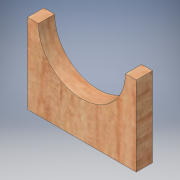
# Autodesk Inventor part: Soporte para Cañón
Saved by Autodesk Inventor 2016 SP2 (Build 200236200, 236)
## iProperties
Created: 2017-06-02
Part Number: Soporte para Cañón
Material: Abedul
Document SubType Name: Modeling
Designer: ssant
Density: 0.512 g/cm^3
Appearance: Abedul - Natural brillo medio
Author: ssant
Autodesk Inventor part; units mm, degrees
ref_plane "YZ Plane" through (0, 0, 0) normal (1, 0, 0) x (0, 1, 0)
ref_plane "XZ Plane" through (0, 0, 0) normal (0, 1, 0) x (-1, 0, 0)
ref_plane "XY Plane" through (0, 0, 0) normal (0, 0, 1) x (1, 0, 0)
sketch "Boceto3" plane through (0, 0, 0) normal (0, 0, 1) x (1, 0, 0)
  line L0 (-30, 22) -> (-30, -22)
  line L1 (-30, -22) -> (30, -22)
  line L2 (30, -22) -> (30, 22)
  line L3 (30, 22) -> (24, 22)
  line L4 (-30, 22) -> (-24, 22)
  arc A0 (-24, 22) -> (24, 22) centre (0, 22) ccw
  point P0 (0, 0)
  point P1 (0, -22)
  point P2 (30, 0)
  dimension "d14" = 44
  dimension "d16" = 60
  dimension "d17" = 44
  dimension "d18" = 6
  dimension "d19" = 6
  dimension "d20" = 90
  dimension "d21" = 48
  constraints: 10 end point, 2 midpoint, 2 perpendicular, 2 point on circle, 1 centre point, 1 horizontal, 1 horizontal alignment, 1 vertical, 1 vertical alignment
  measures "d14" distance of L0.start L0.end
  measures "d16" distance of L0.end L1.end
  measures "d17" distance of L1.end L2.end
  measures "d18" distance of L2.end L3.end
  measures "d19" distance of L0.start L4.end
  measures "d20" angle of L0 L4
  measures "d21" diameter of A0
extrude "Extrusión1" add sketch "Boceto3" against normal blind 9
sketch "Boceto4" plane through (-30, -22, 0) normal (0, -1, 0) x (1, 0, 0)
  line L0 (0, 0) -> (60, 0) projected
  line L1 (0, 0) -> (0, -9) projected
  line L2 (60, -9) -> (0, -9) projected
  line L3 (60, 0) -> (60, -9) projected
  line L4 (60, 0) -> (60, -9) projected
  point P0 (30, 0)
  point P1 (52.5, -4.5)
  point P2 (7.5, -4.5)
  dimension "d26" = 7.5
  dimension "d27" = 4.5
  dimension "d28" = 7.5
  dimension "d29" = 4.5
  measures "d26" distance from line of L3 point (52.5, -4.5)
  measures "d27" distance from line of L2 point (52.5, -4.5)
  measures "d28" distance from line of L1 point (7.5, -4.5)
  measures "d29" distance from line of L2 point (7.5, -4.5)
hole "Agujero1" at (22.5, -22, -4.5) at (-22.5, -22, -4.5) direction (0, 1, 0) diameter 5 depth 20
